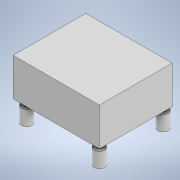
# Autodesk Inventor part: U2D2PHB_Board
Saved by Autodesk Inventor 2022 (Build 260153000, 153)
## iProperties
Created: 2021-09-17
Part Number: U2D2PHB_Board
Material: Generic
Document SubType Name: Modeling
Designer: kylem
Density: 1 g/cm^3
Appearance: Default
Author: kylem
Autodesk Inventor part; units mm, degrees
ref_plane "YZ Plane" through (0, 0, 0) normal (1, 0, 0) x (0, 1, 0)
ref_plane "XZ Plane" through (0, 0, 0) normal (0, 1, 0) x (-1, 0, 0)
ref_plane "XY Plane" through (0, 0, 0) normal (0, 0, 1) x (1, 0, 0)
sketch "Sketch1" plane through (0, 0, 0) normal (0, 1, 0) x (-1, 0, 0)
  line L0 (0, 0) -> (57, 0)
  line L1 (57, 0) -> (57, -48)
  line L2 (57, -48) -> (0, -48)
  line L3 (0, -48) -> (0, 0)
  dimension "d0" = 57
  dimension "d1" = 48
  constraints: 8 end point, 2 parallel, 1 horizontal, 1 perpendicular
  measures "d0" distance of L1.end L2.end
  measures "d1" distance of L0.end L1.end
extrude "Extrusion1" add sketch "Sketch1" along normal blind 25
sketch "Sketch5" plane through (0, 0, 0) normal (0, -1, 0) x (1, 0, 0)
  circle A0 centre (-3, -2.965) radius 1.5 projected
  circle A1 centre (-3, -2.965) radius 3.425
  circle A2 centre (-3, -45.035) radius 1.5 projected
  circle A3 centre (-3, -45.035) radius 3.425
  circle A4 centre (-51.04, -45.035) radius 1.5 projected
  circle A5 centre (-51.04, -45.035) radius 3.425
  circle A6 centre (-51.04, -2.965) radius 1.5 projected
  circle A7 centre (-51.04, -2.965) radius 3.425
  point P0 (0, 0)
  dimension "d19" = 6.85
  dimension "d20" = 6.85
  dimension "d21" = 6.85
  dimension "d22" = 6.85
  constraints: 4 centre point, 4 coincident
  measures "d19" diameter of A1
  measures "d20" diameter of A3
  measures "d21" diameter of A5
  measures "d22" diameter of A7
extrude "Extrusion5" add sketch "Sketch5" along normal blind 12 contours A0 | A1 | A2 | A3 | A4 | A5 | A6 | A7
sketch "Sketch6" plane through (0, 0, 0) normal (0, -1, 0) x (1, 0, 0)
  line L0 (-57, 0) -> (0, 0) projected
  line L1 (0, 0) -> (-57, 0)
  line L2 (-57, -48) -> (-57, 0) projected
  line L3 (-57, 0) -> (-57, -48)
  line L4 (-57, -48) -> (-57, -36.25)
  line L5 (-57, -36.25) -> (-60.9, -36.25)
  line L6 (-60.9, -36.25) -> (-60.9, -27.25)
  line L7 (-60.9, -27.25) -> (-57, -27.25)
  dimension "d25" = 11.75
  dimension "d26" = 3.9
  dimension "d27" = 9
  constraints: 12 end point, 3 perpendicular, 2 point on line, 1 collinear, 1 horizontal
  measures "d25" distance of L2.start L4.end
  measures "d26" distance of L4.end L5.end
  measures "d27" distance of L5.end L6.end
extrude "Extrusion6" add sketch "Sketch6" against normal blind 12.6
sketch "Sketch7" plane through (0, 0, 0) normal (0, -1, 0) x (1, 0, 0)
  line L0 (-60.9, -27.25) -> (-60.9, -36.25) projected
  line L1 (-60.9, -36.25) -> (-57, -36.25)
  line L2 (-57, -36.25) -> (-57, -27.25)
  line L3 (-57, -27.25) -> (-60.9, -27.25)
  line L4 (-60.9, -27.25) -> (-60.9, -36.25)
  point P0 (0, 0)
  constraints: 8 end point, 2 parallel, 1 horizontal, 1 perpendicular
extrude "Extrusion7" cut sketch "Sketch7" against normal blind 1.6
sketch "Sketch8" plane through (-60.9, 12.6, -36.25) normal (-1, 0, 0) x (0, 0, 1)
  line L0 (0, -11) -> (0, 0) projected
  line L1 (0, -11) -> (0, -7.7)
  line L2 (0, -7.7) -> (9, -7.7)
  line L3 (9, 0) -> (9, -11) projected
  line L4 (4.5, -7.7) -> (4.5, -4.95)
  circle A0 centre (4.5, -4.95) radius 2.75
  point P0 (36.25, -12.6)
  dimension "d32" = 3.3
  dimension "d33" = 2.75
  dimension "d34" = 5.5
  constraints: 6 end point, 2 point on line, 1 centre point, 1 coincident, 1 midpoint, 1 perpendicular, 1 vertical
  measures "d32" distance of L0.start L1.end
  measures "d33" distance of L4.start L4.end
  measures "d34" diameter of A0
extrude "Extrusion8" cut sketch "Sketch8" against normal blind 11
sketch "Sketch9" plane through (-3, -12, -45.035) normal (0, -1, 0) x (1, 0, 0)
  circle A0 centre (0, 0) radius 1.5 projected
  circle A1 centre (0, 0) radius 1.5
  circle A2 centre (-48.04, 0) radius 1.5 projected
  circle A3 centre (-48.04, 0) radius 1.5
  arc A4 (-1.7145, 45.035) -> (3, 40.4175) centre (0, 42.07) ccw projected
  circle A5 centre (0, 42.07) radius 1.5
  circle A6 centre (-48.04, 42.07) radius 3.425 projected
  circle A7 centre (-48.04, 42.07) radius 1.5
  point P0 (3, 45.035)
  dimension "d37" = 3
  dimension "d38" = 3
  dimension "d39" = 3
  dimension "d40" = 3
  constraints: 4 centre point, 4 coincident
  measures "d37" diameter of A1
  measures "d38" diameter of A3
  measures "d39" diameter of A5
  measures "d40" diameter of A7
extrude "Extrusion9" cut sketch "Sketch9" against normal blind 10 contours A0 | A2 | A5 | A7
sketch "Sketch10" plane through (0, 0, 0) normal (0, -1, 0) x (1, 0, 0)
  circle A0 centre (-3, -2.965) radius 1.5 projected
  circle A1 centre (-3, -2.965) radius 3.425
  circle A2 centre (-3, -45.035) radius 1.5 projected
  circle A3 centre (-3, -45.035) radius 3.7391
  arc A4 (-49.3255, -48) -> (-52.7545, -48) centre (-51.04, -45.035) ccw projected
  circle A5 centre (-51.04, -45.035) radius 4.1753
  circle A6 centre (-51.04, -2.965) radius 1.5 projected
  circle A7 centre (-51.04, -2.965) radius 4.4366
  point P0 (0, 0)
  constraints: 4 centre point, 4 coincident
extrude "Extrusion10" cut sketch "Sketch10" along normal blind 2 contours A0 | A1 | A2 | A3 | A5 | A6 | A7
body "Solid1"
